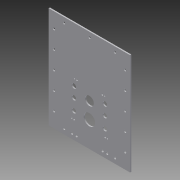
# Autodesk Inventor part: CustomAM-2230
Saved by Autodesk Inventor 2013 (Build 170138000, 138)
## iProperties
Created: 2013-01-23
Part Number: CustomAM-2230
Material: Generic
Document SubType Name: Modeling
Designer: carneeki
Density: 1 g/cm^3
Author: carneeki
Autodesk Inventor part; units mm, degrees
ref_plane "YZ Plane" through (0, 0, 0) normal (1, 0, 0) x (0, 1, 0)
ref_plane "XZ Plane" through (0, 0, 0) normal (0, 1, 0) x (-1, 0, 0)
ref_plane "XY Plane" through (0, 0, 0) normal (0, 0, 1) x (1, 0, 0)
sketch "Sketch1" plane through (0, 0, 0) normal (0, 0, 1) x (1, 0, 0)
  line L0 (0, 0) -> (203.2, 0)
  line L1 (101.6, 152.4) -> (101.6, 0) construction
  circle A0 centre (57.8358, 12.7) radius 3.3528
  circle A1 centre (69.088, 12.7) radius 3.3528
  circle A2 centre (57.023, 45.1866) radius 2.032
  circle A3 centre (62.865, 45.1866) radius 2.54
  circle A4 centre (62.865, 63.5) radius 5.5626
  line L2 (62.865, 0) -> (62.865, 138.1252) construction
  circle A5 centre (62.865, 91.6686) radius 5.5626
  circle A6 centre (62.865, 117.0686) radius 5.5626
  circle A7 centre (69.85, 134.0866) radius 2.54
  circle A8 centre (64.008, 134.0866) radius 2.032
  circle A9 centre (101.6, 63.5) radius 14.2875
  circle A10 centre (101.6, 104.2162) radius 11.1125
  line L3 (0, 0) -> (0, 254) construction
  line L4 (203.2, 0) -> (203.2, 254) construction
  line L5 (0, 254) -> (203.2, 254) construction
  line L6 (120.9294, 254) -> (124.1044, 254) construction
  circle A11 centre (145.3642, 12.7) radius 3.3528
  circle A12 centre (134.112, 12.7) radius 3.3528
  circle A13 centre (146.177, 45.1866) radius 2.032
  circle A14 centre (140.335, 45.1866) radius 2.54
  circle A15 centre (140.335, 63.5) radius 5.5626
  line L7 (140.335, 0) -> (140.335, 138.1252) construction
  circle A16 centre (140.335, 91.6686) radius 5.5626
  circle A17 centre (140.335, 117.0686) radius 5.5626
  circle A18 centre (133.35, 134.0866) radius 2.54
  circle A19 centre (139.192, 134.0866) radius 2.032
  line L8 (0, 254) -> (0, 0)
  line L9 (0, 254) -> (203.2, 254)
  line L10 (203.2, 254) -> (203.2, 0)
  line L11 (57.8358, 12.7) -> (145.3642, 12.7) construction
  line L12 (57.023, 45.1866) -> (146.177, 45.1866) construction
  line L13 (38.1, 241.3) -> (165.1, 241.3) construction
  line L14 (165.1, 241.3) -> (165.1, 12.7) construction
  line L15 (165.1, 12.7) -> (38.1, 12.7) construction
  line L16 (38.1, 12.7) -> (38.1, 241.3) construction
  line L17 (12.7, 215.9) -> (190.5, 215.9) construction
  line L18 (190.5, 215.9) -> (190.5, 38.1) construction
  line L19 (190.5, 38.1) -> (12.7, 38.1) construction
  line L20 (12.7, 38.1) -> (12.7, 215.9) construction
  circle A20 centre (38.1, 241.3) radius 3.175
  circle A21 centre (165.1, 241.3) radius 3.175
  circle A22 centre (190.5, 215.9) radius 3.175
  circle A23 centre (12.7, 215.9) radius 3.175
  circle A24 centre (12.7, 38.1) radius 3.175
  circle A25 centre (38.1, 12.7) radius 3.175
  circle A26 centre (165.1, 12.7) radius 3.175
  circle A27 centre (190.5, 38.1) radius 3.175
  line L21 (0, 127) -> (203.2, 127) construction
  circle A28 centre (12.7, 127) radius 3.175
  circle A29 centre (190.5, 127) radius 3.175
  circle A30 centre (101.6, 241.3) radius 3.175
  circle A31 centre (12.7, 171.45) radius 3.175
  circle A32 centre (12.7, 82.55) radius 3.175
  circle A33 centre (190.5, 82.55) radius 3.175
  circle A34 centre (190.5, 171.45) radius 3.175
  point P0 (140.335, 69.0626)
  dimension "d115" = 254
  dimension "d116" = 203.2
  dimension "d130" = 77.47
  dimension "d131" = 38.735
  dimension "d133" = 31.75
  dimension "d134" = 37.592
  dimension "d135" = 38.735
  dimension "d138" = 38.735
  dimension "d149" = 12.7
  dimension "d150" = 5.08
  dimension "d151" = 4.064
  dimension "d152" = 11.1252
  dimension "d153" = 22.225
  dimension "d155" = 6.7056
  dimension "d183" = 79.0956
  dimension "d184" = 82.2706
  dimension "d185" = 101.6
  dimension "d189" = 12.7
  dimension "d190" = 38.1
  dimension "d191" = 38.1
  dimension "d192" = 12.7
  dimension "d193" = 38.1
  dimension "d194" = 12.7
  dimension "d195" = 12.7
  dimension "d196" = 38.1
  dimension "d197" = 6.35
  dimension "d198" = 6.35
  dimension "d199" = 6.35
  dimension "d200" = 6.35
  dimension "d201" = 6.35
  dimension "d202" = 6.35
  dimension "d203" = 6.35
  dimension "d204" = 6.35
  dimension "d205" = 6.35
  dimension "d206" = 6.35
  dimension "d207" = 6.35
  dimension "d213" = 6.35
  dimension "d216" = 6.35
  dimension "d218" = 6.35
  dimension "d220" = 6.35
  dimension "d225" = 177.8
  dimension "d226" = 44.45
  dimension "d227" = 44.45
  dimension "d228" = 44.45
  dimension "d229" = 44.45
  dimension "d230" = 44.45
  dimension "d231" = 44.45
  dimension "d241" = 63.5
  dimension "d242" = 40.7162
  dimension "d250" = 18.3134
  dimension "d251" = 25.4
  dimension "d252" = 17.018
  dimension "d256" = 63.5
  constraints: 44 end point, 34 centre point, 11 symmetric about line, 8 coincident, 8 point on line, 7 midpoint, 7 parallel, 6 perpendicular, 5 equal radius, 5 horizontal alignment, 4 horizontal, 3 vertical alignment, 1 vertical, 11 other
  measures "d115" distance of L3.end L0.start
  measures "d116" distance of L0.start L0.end
  measures "d130" distance between parallel lines of L7 L2
  measures "d131" distance between parallel lines of L1 L7
  measures "d133" distance from line of L1 A7.centre
  measures "d134" distance from line of A8.centre L1
  measures "d135" distance from line of A6.centre L1
  measures "d138" distance between parallel lines of L2 L1
  measures "d149" distance between parallel lines of L0 L11
  measures "d150" diameter of A7
  measures "d151" diameter of A8
  measures "d152" diameter of A6
  measures "d153" diameter of A10
  measures "d155" diameter of A0
  measures "d183" distance from line of L6.end L10
  measures "d184" distance from line of L6.start L10
  measures "d185" distance from line of L1.start L6
  measures "d189" distance between parallel lines of L5 L13
  measures "d190" distance between parallel lines of L8 L16
  measures "d191" distance between parallel lines of L10 L14
  measures "d192" distance between parallel lines of L0 L15
  measures "d193" distance between parallel lines of L5 L17
  measures "d194" distance between parallel lines of L3 L20
  measures "d195" distance between parallel lines of L10 L18
  measures "d196" distance between parallel lines of L0 L19
  measures "d197" diameter of A20
  measures "d198" diameter of A21
  measures "d199" diameter of A22
  measures "d200" diameter of A23
  measures "d201" diameter of A24
  measures "d202" diameter of A25
  measures "d203" diameter of A26
  measures "d204" diameter of A27
  measures "d205" diameter of A28
  measures "d206" diameter of A29
  measures "d207" diameter of A30
  measures "d213" diameter of A31
  measures "d216" diameter of A32
  measures "d218" diameter of A33
  measures "d220" diameter of A34
  measures "d225" distance of L19.end L17.start
  measures "d226" distance of L19.end A32.centre
  measures "d227" distance of A32.centre A28.centre
  measures "d228" distance of A28.centre A31.centre
  measures "d229" distance of A29.centre A34.centre
  measures "d230" distance of A29.centre A33.centre
  measures "d231" distance of L18.end A33.centre
  measures "d241" distance from line of L0 A9.centre
  measures "d242" distance of A9.centre A10.centre
  measures "d250" vertical distance of A3.centre A9.centre
  measures "d251" distance of A5.centre A6.centre
  measures "d252" vertical distance of A6.centre A7.centre
  measures "d256" distance from line of A4.centre L0
extrude "Extrusion2" add sketch "Sketch1" along normal blind 3
equation "\"d191\" = d190"
equation "\"d192\" = d189"
equation "\"d193\" = d190"
equation "\"d194\" = d189"
equation "\"d195\" = d189"
equation "\"d196\" = d190"
equation "\"d226\" = 0.25 * d225"
equation "\"d228\" = 0.25 * d225"
equation "\"d229\" = d226"
equation "\"d230\" = d226"
body "Solid2"
